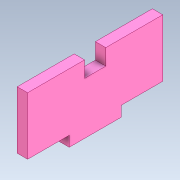
# Autodesk Inventor part: BackWall
Saved by Autodesk Inventor 2021 (Build 250183000, 183)
## iProperties
Created: 2021-08-31
Part Number: BackWall
Material: ABS Plastic
Document SubType Name: Modeling
Designer: digge
Density: 1.06 g/cm^3
Appearance: Pink
Author: digge
Autodesk Inventor part; units mm, degrees
ref_plane "YZ Plane" through (0, 0, 0) normal (1, 0, 0) x (0, 1, 0)
ref_plane "XZ Plane" through (0, 0, 0) normal (0, 1, 0) x (-1, 0, 0)
ref_plane "XY Plane" through (0, 0, 0) normal (0, 0, 1) x (1, 0, 0)
sketch "Sketch1" plane through (0, 0, 0) normal (1, 0, 0) x (0, 1, 0)
  line L0 (104.8505, 212.4728) -> (49.4505, 212.4728)
  line L1 (49.4505, 212.4728) -> (49.4505, 172.4728)
  line L2 (49.4505, 122.4728) -> (49.4505, 82.4728)
  line L3 (49.4505, 82.4728) -> (104.8505, 82.4728)
  line L4 (104.8505, 82.4728) -> (104.8505, 137.2728)
  line L5 (104.8505, 137.2728) -> (89.4505, 137.2728)
  line L6 (89.4505, 137.2728) -> (89.4505, 157.6728)
  line L7 (89.4505, 157.6728) -> (104.8505, 157.6728)
  line L8 (104.8505, 212.4728) -> (104.8505, 157.6728)
  line L9 (39.4505, 147.4728) -> (89.4505, 147.4728) construction
  line L10 (39.4505, 172.4728) -> (39.4505, 122.4728)
  line L11 (49.4505, 122.4728) -> (39.4505, 122.4728)
  line L12 (49.4505, 172.4728) -> (39.4505, 172.4728)
  point P0 (0, 0)
  dimension "d0" = 10
  dimension "d3" = 55.4
  dimension "d4" = 130
  dimension "d8" = 20.4
  dimension "d9" = 50
  dimension "d10" = 15.4
  constraints: 26 end point, 5 perpendicular, 2 horizontal, 2 point on line, 1 midpoint, 1 parallel, 1 vertical, 2 other
  measures "d0" distance of L1.end L10.start
  measures "d3" distance of L0.start L0.end
  measures "d4" distance between parallel lines of L3 L0
  measures "d8" distance of L5.end L6.end
  measures "d9" distance of L10.start L10.end
  measures "d10" distance of L6.end L7.end
extrude "Extrusion1" add sketch "Sketch1" along normal blind 10
equation "\"d0\" = Width"
equation "\"d5\" = Width"
equation "\"Width\" = 10"
body "Solid1"
